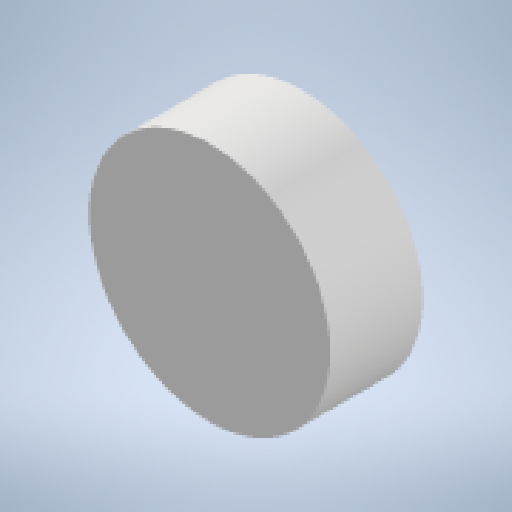
# Autodesk Inventor part: LeftEyePeach
Saved by Autodesk Inventor 2023 (Build 270158000, 158)
## iProperties
Created: 2022-11-09
Part Number: LeftEyePeach
Material: Generic
Document SubType Name: Modeling
Designer: reide
Density: 1 g/cm^3
Appearance: Default
Author: reide
Autodesk Inventor part; units mm, degrees
ref_plane "YZ Plane" through (0, 0, 0) normal (1, 0, 0) x (0, 1, 0)
ref_plane "XZ Plane" through (0, 0, 0) normal (0, 1, 0) x (-1, 0, 0)
ref_plane "XY Plane" through (0, 0, 0) normal (0, 0, 1) x (1, 0, 0)
sketch "Sketch1" plane through (0, 0, 0) normal (0, 0, 1) x (1, 0, 0)
  arc A0 (-2.66, 28.9502) -> (-6.8568, 25.0691) centre (-1.7554, 23.7624) ccw projected
  ellipse E0 centre (-11.6202, 25.5) end of major axis (-16.3836, 25.9309) minor radius 4.1297 (-6.983, 24.3981) -> (-6.8568, 25.0691) ccw projected
  arc A1 (-6.8568, 25.0691) -> (-6.983, 24.3981) centre (-1.7554, 23.7624) ccw projected
  ellipse E1 centre (-11.6202, 25.5) end of major axis (-6.8568, 25.0691) minor radius 4.1297 (-6.8568, 25.0691) -> (-9.0924, 28.9502) ccw projected
  line L0 (-2.66, 28.9502) -> (-9.0924, 28.9502) projected
  arc A2 (-61.3309, 28.9502) -> (-62.6675, 26.9113) centre (-44.0465, 16.1615) ccw projected
  spline S0 degree 3 poles (-58.653, 25.192) (-58.6606, 25.1631) (-58.6686, 25.1343) (-58.7991, 24.6877) (-59.003, 24.2939) (-59.4852, 23.6838) (-59.7387, 23.4471) (-60.2828, 23.092) (-60.5675, 22.9639) (-61.1231, 22.8345) (-61.3904, 22.8182) (-61.8134, 22.8805) (-61.973, 22.9257) (-62.1234, 22.9922) (-62.4076, 23.1178) (-62.656, 23.3208) (-62.9477, 23.7101) (-63.0339, 23.8647) (-63.2588, 24.4075) (-63.3118, 24.8274) (-63.242, 25.7644) (-63.0671, 26.2783) (-62.751, 26.7899) (-62.7103, 26.8512) (-62.6675, 26.9113) knots -2.04297 -2.04297 -2.04297 -2.04297 -2.033998 -2.033998 -1.903383 -1.903383 -1.8007 -1.8007 -1.70847 -1.70847 -1.629539 -1.629539 -1.580207 -1.580207 -1.580207 -1.486994 -1.486994 -1.434286 -1.434286 -1.31073 -1.31073 -1.152429 -1.152429 -1.130329 -1.130329 -1.130329 -1.130329 projected
  arc A3 (-55.7904, 28.9502) -> (-58.653, 25.192) centre (-50.9143, 22.2669) ccw projected
  line L1 (-50.5459, 28.9502) -> (-55.7904, 28.9502) projected
  arc A4 (-50.5459, 28.9502) -> (-46.1154, 25.1531) centre (-37.1131, 40.1401) ccw projected
  arc A5 (-46.1154, 25.1531) -> (-55.0724, 17.1262) centre (-42.6959, 12.3264) ccw projected
  arc A6 (-55.0724, 17.1262) -> (-56.9124, 0.0781) centre (-27.25, 5.5) ccw projected
  arc A7 (-56.9124, 0.0781) -> (-63.9254, -11.1644) centre (-45.9, -14.6) ccw projected
  arc A8 (-63.9254, -11.1644) -> (-50.5956, -15.4346) centre (-53, 0) ccw projected
  arc A9 (-50.5956, -15.4346) -> (-5.024, -24.0976) centre (-22.4792, 8.2756) ccw projected
  arc A10 (-5.024, -24.0976) -> (8.0763, -24.7873) centre (2.3257, -9.2566) ccw projected
  arc A11 (8.0763, -24.7873) -> (5.2801, -14.6676) centre (-6.5408, -23.3801) ccw projected
  arc A12 (5.2801, -14.6676) -> (7.9552, -1.1219) centre (-13.9278, -3.8373) ccw projected
  arc A13 (7.9552, -1.1219) -> (1.4312, 20.9259) centre (-1.7554, 7.9938) ccw projected
  arc A14 (1.4312, 20.9259) -> (-0.9419, 27.9502) centre (-1.7554, 23.7624) ccw projected
  line L2 (-0.9419, 27.9502) -> (0.4374, 27.9502) projected
  arc A15 (1.4374, 28.9502) -> (0.4374, 27.9502) centre (1.4374, 27.9502) ccw projected
  line L3 (68.6006, 28.9502) -> (1.4374, 28.9502) projected
  line L4 (68.6006, 36.9518) -> (68.6006, 28.9502) projected
  line L5 (-63.1756, 36.9518) -> (68.6006, 36.9518) projected
  arc A16 (-65.1756, 38.9518) -> (-63.1756, 36.9518) centre (-63.1756, 38.9518) ccw projected
  line L6 (-65.1756, 131.9502) -> (-65.1756, 38.9518) projected
  arc A17 (-63.1756, 133.9502) -> (-65.1756, 131.9502) centre (-63.1756, 131.9502) ccw projected
  line L7 (68.6006, 133.9502) -> (-63.1756, 133.9502) projected
  line L8 (68.6006, 141.9502) -> (68.6006, 133.9502) projected
  line L9 (-68.6006, 141.9502) -> (68.6006, 141.9502) projected
  arc A18 (-68.6006, 141.9502) -> (-72.6006, 137.9502) centre (-68.6006, 137.9502) ccw projected
  line L10 (-72.6006, 32.9502) -> (-72.6006, 137.9502) projected
  arc A19 (-72.6006, 32.9502) -> (-68.6006, 28.9502) centre (-68.6006, 32.9502) ccw projected
  line L11 (-61.3309, 28.9502) -> (-68.6006, 28.9502) projected
  ellipse E2 centre (-12.4142, 25.5) end of major axis (-16.852, 25.5) minor radius 3.9921 projected
  ellipse E3 centre (-29, 6.4502) end of major axis (-32, 6.4502) minor radius 2.4928 projected
  arc A20 (-56.1817, -1.6982) -> (-51.5706, -13.5582) centre (83.9158, 45.9447) ccw projected
  arc A21 (-61.7014, -10.3098) -> (-51.5706, -13.5582) centre (-51.0305, 5.5476) ccw projected
  arc A22 (-56.1817, -1.6982) -> (-61.7014, -10.3098) centre (-43.1644, -16.1163) ccw projected
  arc A23 (-7.3959, 3.4823) -> (-9, 2.4502) centre (-7.6242, 2.0744) ccw projected
  arc A24 (-9, 2.4502) -> (-10.9261, 4.4246) centre (-12, 1.4502) ccw projected
  ellipse E4 centre (-9.1559, 4.4502) end of major axis (-9.1559, 13.4502) minor radius 1.7702 (-7.3959, 3.4823) -> (-10.9261, 4.4246) ccw projected
  circle A25 centre (0, 0) radius 2.7388 projected
  circle A26 centre (-22, 1.4502) radius 2.8284 projected
  arc A27 (-0.8225, -23.5484) -> (5.4696, -17.745) centre (-15.1533, -1.6982) ccw projected
  arc A28 (5.9278, -23.467) -> (5.4696, -17.745) centre (-12.2658, -22.0444) ccw projected
  arc A29 (-0.8225, -23.5484) -> (5.9278, -23.467) centre (2.3663, -8.0668) ccw projected
  ellipse E5 centre (-1.7554, 24.0133) end of major axis (2.2633, 23.7374) minor radius 3.5714 projected
  ellipse E6 centre (6.4561, 3.1917) end of major axis (3.9246, 3.1917) minor radius 2.1289 projected
  circle A30 centre (0, 0) radius 2.6019
  constraints: 1 centre point, 1 coincident, 6 other
extrude "Extrusion1" add sketch "Sketch1" along normal blind 2 contours A30
body "Solid1"
